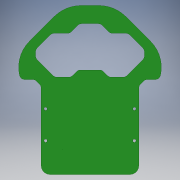
# Autodesk Inventor part: mainpcb
Saved by Autodesk Inventor 2016 (Build 200138000, 138)
## iProperties
Created: 2017-05-27
Part Number: mainpcb
Material: Ogólny
Document SubType Name: Modeling
Designer: Karol
Density: 1 g/cm^3
Appearance: Smooth - Dark Forest Green
Author: Karol
Autodesk Inventor part; units mm, degrees
ref_plane "YZ Plane" through (0, 0, 0) normal (1, 0, 0) x (0, 1, 0)
ref_plane "XZ Plane" through (0, 0, 0) normal (0, 1, 0) x (-1, 0, 0)
ref_plane "XY Plane" through (0, 0, 0) normal (0, 0, 1) x (1, 0, 0)
sketch "Sketch1" plane through (0, 0, 0) normal (0, 1, 0) x (-1, 0, 0)
  line L0 (0, 0) -> (0, 22.5)
  line L1 (5, 27.5) -> (48.7574, 27.5)
  arc A0 (5, 27.5) -> (0, 22.5) centre (5, 22.5) ccw
  arc A1 (95.1955, 5) -> (89.1353, 20) centre (73.6017, 5) ccw
  line L2 (89.1353, 20) -> (74.9931, 34.1421)
  line L3 (26, 0) -> (39.959, 0)
  line L4 (95.1955, 5) -> (95.1955, 0)
  line L5 (0, 0) -> (0, -22.5)
  arc A2 (0, -22.5) -> (5, -27.5) centre (5, -22.5) ccw
  line L6 (50.8787, 28.3787) -> (52.6569, 30.1569)
  line L7 (53.5355, 32.2782) -> (53.5355, 36.7771)
  arc A3 (74.9931, 34.1421) -> (55.8844, 39.7056) centre (60.372, 19.521) ccw
  line L8 (55.7045, 20.8787) -> (64.6301, 29.805)
  line L9 (66.7515, 30.6838) -> (69.1812, 30.6838)
  arc A4 (71.3025, 29.8051) -> (69.1812, 30.6838) centre (69.1812, 27.6838) ccw
  arc A5 (66.7515, 30.6838) -> (64.6301, 29.805) centre (66.7515, 27.6838) ccw
  arc A6 (55.7045, 20.8787) -> (54.8259, 18.7574) centre (57.8259, 18.7574) ccw
  arc A7 (48.7574, 27.5) -> (50.8787, 28.3787) centre (48.7574, 30.5) ccw
  arc A8 (52.6569, 30.1569) -> (53.5355, 32.2782) centre (50.5355, 32.2782) ccw
  arc A9 (55.8844, 39.7056) -> (53.5355, 36.7771) centre (56.5355, 36.7771) ccw
  arc A10 (89.1353, -20) -> (95.1955, -5) centre (73.6017, -5) ccw
  line L10 (89.1353, -20) -> (74.9931, -34.1421)
  line L11 (95.1955, -5) -> (95.1955, 0)
  line L12 (50.8787, -28.3787) -> (52.6569, -30.1569)
  line L13 (53.5355, -32.2782) -> (53.5355, -36.7771)
  arc A11 (55.8844, -39.7056) -> (74.9931, -34.1421) centre (60.372, -19.521) ccw
  arc A12 (50.8787, -28.3787) -> (48.7574, -27.5) centre (48.7574, -30.5) ccw
  arc A13 (53.5355, -32.2782) -> (52.6569, -30.1569) centre (50.5355, -32.2782) ccw
  arc A14 (53.5355, -36.7771) -> (55.8844, -39.7056) centre (56.5355, -36.7771) ccw
  line L14 (48.7574, -27.5) -> (5, -27.5)
  line L15 (71.3025, 29.8051) -> (77.4646, 23.642)
  line L16 (54.8259, 18.7574) -> (54.8259, 11.8995)
  line L17 (55.7046, 9.7782) -> (57.9473, 7.5354)
  line L18 (58.826, 5.4141) -> (58.826, 0)
  arc A15 (54.8259, 11.8995) -> (55.7046, 9.7782) centre (57.8259, 11.8995) ccw
  arc A16 (58.826, 5.4141) -> (57.9473, 7.5354) centre (55.826, 5.4141) ccw
  line L19 (77.4646, 23.642) -> (78.7073, 22.3992)
  line L20 (85, 0) -> (85, 4.757)
  line L21 (84.1209, 6.8787) -> (80.4649, 10.5334)
  line L22 (79.5858, 12.6551) -> (79.5858, 20.2781)
  arc A17 (79.5858, 20.2781) -> (78.7073, 22.3992) centre (76.5858, 20.2781) ccw
  arc A18 (79.5858, 12.6551) -> (80.4649, 10.5334) centre (82.5858, 12.6551) ccw
  arc A19 (85, 4.757) -> (84.1209, 6.8787) centre (82, 4.757) ccw
  line L23 (55.7045, -20.8787) -> (64.6301, -29.805)
  line L24 (66.7515, -30.6838) -> (69.1812, -30.6838)
  arc A20 (69.1812, -30.6838) -> (71.3025, -29.8051) centre (69.1812, -27.6838) ccw
  arc A21 (64.6301, -29.805) -> (66.7515, -30.6838) centre (66.7515, -27.6838) ccw
  arc A22 (54.8259, -18.7574) -> (55.7045, -20.8787) centre (57.8259, -18.7574) ccw
  line L25 (71.3025, -29.8051) -> (77.4646, -23.642)
  line L26 (54.8259, -18.7574) -> (54.8259, -11.8995)
  line L27 (55.7046, -9.7782) -> (57.9473, -7.5354)
  line L28 (58.826, -5.4141) -> (58.826, 0)
  arc A23 (55.7046, -9.7782) -> (54.8259, -11.8995) centre (57.8259, -11.8995) ccw
  arc A24 (57.9473, -7.5354) -> (58.826, -5.4141) centre (55.826, -5.4141) ccw
  line L29 (77.4646, -23.642) -> (78.7073, -22.3992)
  line L30 (85, 0) -> (85, -4.757)
  line L31 (84.1209, -6.8787) -> (80.4649, -10.5334)
  line L32 (79.5858, -12.6551) -> (79.5858, -20.2781)
  arc A25 (78.7073, -22.3992) -> (79.5858, -20.2781) centre (76.5858, -20.2781) ccw
  arc A26 (80.4649, -10.5334) -> (79.5858, -12.6551) centre (82.5858, -12.6551) ccw
  arc A27 (84.1209, -6.8787) -> (85, -4.757) centre (82, -4.757) ccw
  point P0 (0, 27.5)
  point P1 (80, 0)
  point P2 (42, 25)
  point P3 (14, 25)
  point P4 (14, 15.5)
  point P5 (37, 25)
  point P6 (19, 25)
  point P7 (0, -27.5)
  point P8 (42, -25)
  point P9 (14, -25)
  point P10 (14, -15.5)
  point P11 (37, -25)
  point P12 (19, -25)
  point P13 (53.5355, 31.0355)
  point P14 (53.5355, 39.0355)
  point P15 (70.4238, 30.6838)
  point P16 (86.6252, 0)
  point P17 (54.8259, 20)
  point P18 (65.5088, 30.6838)
  point P19 (53.5355, -31.0355)
  point P20 (53.5355, -39.0355)
  point P21 (78.3431, 10.6569)
  point P22 (79.5858, 21.5206)
  point P23 (85, 6)
  point P24 (79.5858, 11.4122)
  point P25 (78.3431, -10.6569)
  point P26 (85, -6)
  point P27 (79.5858, -11.4122)
  dimension "d2" = 27.5
  dimension "d19" = 5
  dimension "d43" = 28
  dimension "d45" = 12
  dimension "d73" = 20
  dimension "d118" = 8
  dimension "d124" = 3
  dimension "d125" = 3
  dimension "d126" = 3
  dimension "d127" = 3
  dimension "d128" = 3
  dimension "d129" = 3
  dimension "d133" = 14
  dimension "d140" = 3
  dimension "d141" = 3
  dimension "d143" = 6
  dimension "d144" = 3
  constraints: 66 end point, 66 symmetric about line, 58 point on circle, 28 centre point, 24 tangent, 23 point on line, 7 vertical, 4 horizontal, 3 equal radius, 14 other
  measures "d2" distance of L0.start point (0, 27.5)
  measures "d19" radius of A0
  measures "d43" distance of point (14, 25) point (42, 25)
  measures "d45" distance from line of L1 point (14, 15.5)
  measures "d73" distance of L2.start L2.end
  measures "d118" distance of point (53.536, 31.036) point (53.536, 39.036)
  measures "d124" radius of A4
  measures "d125" radius of A5
  measures "d126" radius of A6
  measures "d127" radius of A7
  measures "d128" radius of A8
  measures "d129" radius of A9
  measures "d133" distance from line of L0 point (14, 15.5)
  measures "d140" radius of A15
  measures "d141" distance of L15.end point (79.586, 21.521)
  measures "d143" distance of L20.start point (85, 6)
  measures "d144" radius of A17
extrude "Extrusion1" add sketch "Sketch1" along normal blind 1.4
hole "Hole1" at (-37, 0, 25) at (-19, 0, 25) at (-37, 0, -25) at (-19, 0, -25) direction (0, 1, 0) diameter 2 depth 2 tip angle 118
hole "Hole3" at (-14, 0, 15.5) direction (0, 1, 0) diameter 0.1 depth 8 tip angle 118
body "Solid1"
